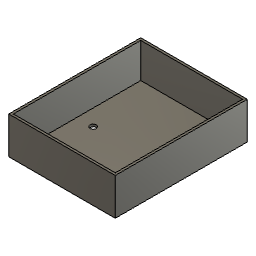
Battery Case (Autodesk Fusion 360 design; units mm, degrees)
Autodesk Fusion 360 part; units mm, degrees
sketch "Sketch1" plane through (0, 0, 0) normal (0, 1, 0) x (1, 0, 0)
  line L0 (0, 0) -> (46, 0)
  line L1 (46, 0) -> (46, -57)
  line L2 (46, -57) -> (0, -57)
  line L3 (0, -57) -> (0, 0)
  dimension "d1" = 46
  dimension "d2" = 57
  constraint horizontal L0
  constraint vertical L1
  constraint horizontal L2
  constraint vertical L3
  constraint coincident L0.start L3.end
  measures "d1" distance of L0.start L0.end
  measures "d2" distance of L0.start L2.end
extrude "Extrude1" add sketch "Sketch1" along normal blind 16
shell "Shell1" thickness 1 removed faces 1 at (15.3333, 16, 19)
move_body "Move1" bodies 1 to x (1, 0, 0) y (0, 1, 0) z (0, 0, 1) at (-23, 15, -28.5)
move_body "Move2" bodies 1 to x (1, 0, 0) y (0, 1, 0) z (0, 0, 1) at (0, -15, 0)
sketch "Sketch2" plane through (0, 1, 0) normal (0, 1, 0) x (-1, 0, 0)
  line L0 (22, 27.5) -> (-22, 27.5)
  line L1 (-22, 27.5) -> (-22, -27.5)
  line L2 (-22, -27.5) -> (22, -27.5)
  line L3 (22, -27.5) -> (22, 27.5)
  circle A0 centre (15, 0) radius 1.35
  circle A1 centre (-15, 0) radius 1.35
  line L4 (23, 0) -> (-23, 0) construction
  dimension "d6" = 2.7
  dimension "d7" = 2.7
  dimension "d8" = 8
  dimension "d9" = 8
  constraint perpendicular L1 L4
  constraint coincident A0.centre L4
  constraint coincident A1.centre L4
  measures "d6" diameter of A0
  measures "d7" diameter of A1
  measures "d8" distance of A0.centre L4.start
  measures "d9" distance of A1.centre L4.end
extrude "Extrude2" cut sketch "Sketch2" against normal up to surface (1 mm away) contours A0 | A1
